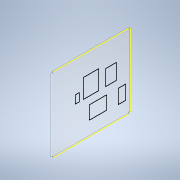
# Autodesk Inventor part: BackMountingWall
Saved by Autodesk Inventor 2020 (Build 240168000, 168)
## iProperties
Created: 2020-04-20
Part Number: BackMountingWall
Material: Типовые
Document SubType Name: Modeling
Designer: Михаил
Density: 1 g/cm^3
Appearance: По умолчанию
Author: Михаил
Autodesk Inventor part; units mm, degrees
ref_plane "YZ Plane" through (0, 0, 0) normal (1, 0, 0) x (0, 1, 0)
ref_plane "XZ Plane" through (0, 0, 0) normal (0, 1, 0) x (-1, 0, 0)
ref_plane "XY Plane" through (0, 0, 0) normal (0, 0, 1) x (1, 0, 0)
sketch "Эскиз1" plane through (0, 0, 0) normal (1, 0, 0) x (0, 1, 0)
  line L0 (390, 0) -> (390, -400)
  line L1 (0, -400) -> (0, 0)
  line L2 (385, 8) -> (5, 8)
  line L3 (5, -408) -> (385, -408)
  line L4 (390, 0) -> (385, 0)
  line L5 (385, 8) -> (385, 0)
  line L6 (385, -408) -> (385, -400)
  line L7 (5, -408) -> (5, -400)
  line L8 (5, -400) -> (0, -400)
  line L9 (5, 0) -> (5, 8)
  line L10 (390, -400) -> (385, -400)
  line L11 (5, 0) -> (0, 0)
  dimension "d23" = 400
  dimension "d26" = 400
  dimension "d27" = 380
  dimension "d28" = 380
  dimension "d29" = 390
  dimension "d30" = 8
  dimension "d31" = 8
  dimension "d32" = 8
  dimension "d34" = 5
  dimension "d35" = 5
  dimension "d36" = 5
  dimension "d37" = 5
  constraints: 24 end point, 2 horizontal, 2 parallel, 1 perpendicular, 1 vertical
  measures "d23" distance between parallel lines of L10 L4
  measures "d26" distance of L1.start L1.end
  measures "d27" distance of L2.start L2.end
  measures "d28" distance of L3.start L3.end
  measures "d29" distance of L0.start L1.end
  measures "d30" distance between parallel lines of L2 L11
  measures "d31" distance between parallel lines of L2 L4
  measures "d32" distance between parallel lines of L3 L8
  measures "d34" distance between parallel lines of L1 L9
  measures "d35" distance between parallel lines of L1 L7
  measures "d36" distance between parallel lines of L0 L6
  measures "d37" distance between parallel lines of L0 L5
extrude "Выдавливание1" add sketch "Эскиз1" along normal blind 4
sketch "Эскиз2" plane through (4, 0, 0) normal (1, 0, 0) x (0, 0, -1)
  line L0 (160, 285) -> (240, 285)
  line L1 (240, 285) -> (240, 185)
  line L2 (240, 185) -> (160, 185)
  line L3 (160, 185) -> (160, 285)
  line L4 (117, 227) -> (138, 227)
  line L5 (138, 227) -> (138, 185)
  line L6 (138, 185) -> (117, 185)
  line L7 (117, 185) -> (117, 227)
  line L8 (343, 144) -> (382, 144)
  line L9 (382, 144) -> (382, 70)
  line L10 (382, 70) -> (343, 70)
  line L11 (343, 70) -> (343, 144)
  line L12 (192, 145) -> (282, 145)
  line L13 (282, 145) -> (282, 75)
  line L14 (282, 75) -> (192, 75)
  line L15 (192, 75) -> (192, 145)
  line L16 (277, 267) -> (333, 267)
  line L17 (333, 267) -> (333, 185)
  line L18 (333, 185) -> (277, 185)
  line L19 (277, 185) -> (277, 267)
  line L20 (408, 5) -> (408, 385) projected
  line L21 (0, 0) -> (400, 0) projected
  line L22 (-8, 385) -> (-8, 5) projected
  line L23 (400, 390) -> (0, 390) projected
  dimension "d38" = 42
  dimension "d39" = 21
  dimension "d40" = 74
  dimension "d41" = 39
  dimension "d44" = 90
  dimension "d45" = 70
  dimension "d46" = 80
  dimension "d47" = 100
  dimension "d48" = 82
  dimension "d49" = 56
  dimension "d50" = 65
  dimension "d51" = 70
  dimension "d52" = 200
  dimension "d53" = 75
  dimension "d54" = 168
  dimension "d55" = 105
  dimension "d56" = 185
  dimension "d57" = 125
  dimension "d58" = 185
  dimension "d59" = 75
  constraints: 40 end point, 10 parallel, 5 horizontal, 5 perpendicular
  measures "d38" distance of L6.end L4.start
  measures "d39" distance of L4.start L4.end
  measures "d40" distance of L10.end L8.start
  measures "d41" distance of L8.start L8.end
  measures "d44" distance of L12.start L12.end
  measures "d45" distance of L14.end L12.start
  measures "d46" distance of L0.start L0.end
  measures "d47" distance of L2.end L0.start
  measures "d48" distance of L18.end L16.start
  measures "d49" distance of L16.start L16.end
  measures "d50" distance between parallel lines of L11 L20
  measures "d51" distance between parallel lines of L21 L10
  measures "d52" distance between parallel lines of L22 L15
  measures "d53" distance between parallel lines of L21 L14
  measures "d54" distance between parallel lines of L22 L3
  measures "d55" distance between parallel lines of L23 L0
  measures "d56" distance between parallel lines of L21 L6
  measures "d57" distance between parallel lines of L22 L7
  measures "d58" distance between parallel lines of L21 L18
  measures "d59" distance between parallel lines of L20 L17
